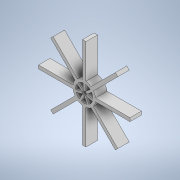
# Autodesk Inventor part: ЛОПАСТИ
Saved by Autodesk Inventor 2020 (Build 240168000, 168)
## iProperties
Created: 2020-09-18
Part Number: ЛОПАСТИ
Material: Типовые
Document SubType Name: Modeling
Designer: uchenik
Density: 1 g/cm^3
Appearance: По умолчанию
Author: uchenik
Autodesk Inventor part; units mm, degrees
ref_plane "YZ Plane" through (0, 0, 0) normal (1, 0, 0) x (0, 1, 0)
ref_plane "XZ Plane" through (0, 0, 0) normal (0, 1, 0) x (-1, 0, 0)
ref_plane "XY Plane" through (0, 0, 0) normal (0, 0, 1) x (1, 0, 0)
sketch "Эскиз1" plane through (0, 0, 0) normal (0, 0, 1) x (1, 0, 0)
  circle A0 centre (0, 0) radius 40
  circle A1 centre (0, 0) radius 10
  circle A2 centre (0, 0) radius 7.5
  line L0 (-1.5, 7.3485) -> (-1.5, 39.9719)
  line L1 (1.5, 7.3485) -> (1.5, 39.9719)
  line L2 (-6.2568, 4.1355) -> (-29.325, 27.2037)
  line L3 (-4.1355, 6.2568) -> (-27.2037, 29.325)
  line L4 (-7.3485, -1.5) -> (-39.9719, -1.5)
  line L5 (-7.3485, 1.5) -> (-39.9719, 1.5)
  line L6 (-4.1355, -6.2568) -> (-27.2037, -29.325)
  line L7 (-6.2568, -4.1355) -> (-29.325, -27.2037)
  line L8 (1.5, -7.3485) -> (1.5, -39.9719)
  line L9 (-1.5, -7.3485) -> (-1.5, -39.9719)
  line L10 (6.2568, -4.1355) -> (29.325, -27.2037)
  line L11 (4.1355, -6.2568) -> (27.2037, -29.325)
  line L12 (7.3485, 1.5) -> (39.9719, 1.5)
  line L13 (7.3485, -1.5) -> (39.9719, -1.5)
  line L14 (4.1355, 6.2568) -> (27.2037, 29.325)
  line L15 (6.2568, 4.1355) -> (29.325, 27.2037)
  circle A3 centre (0, 0) radius 2
  line L16 (-0.8877, 1.7922) -> (-0.8877, 7.4473)
  line L17 (0.8877, 1.7922) -> (0.8877, 7.4473)
  line L18 (-1.9547, 0.4233) -> (-6.376, 3.9492)
  line L19 (-0.8477, 1.8115) -> (-5.269, 5.3374)
  line L20 (-1.5497, -1.2643) -> (-7.063, -2.5227)
  line L21 (-1.9448, 0.4667) -> (-7.4581, -0.7917)
  line L22 (0.0222, -1.9999) -> (-2.4314, -7.0949)
  line L23 (-1.5774, -1.2295) -> (-4.0311, -6.3246)
  line L24 (1.5774, -1.2295) -> (4.0311, -6.3246)
  line L25 (-0.0222, -1.9999) -> (2.4314, -7.0949)
  line L26 (1.9448, 0.4667) -> (7.4581, -0.7917)
  line L27 (1.5497, -1.2643) -> (7.063, -2.5227)
  line L28 (0.8477, 1.8115) -> (5.269, 5.3374)
  line L29 (1.9547, 0.4233) -> (6.376, 3.9492)
  circle A4 centre (-0.0222, 0) radius 1.75
  point P0 (0, 7.5)
  point P1 (-1.5, 9.8869)
  point P2 (-5.9304, 8.0517)
  point P3 (-8.0517, 5.9304)
  point P4 (-9.8869, 1.5)
  point P5 (-9.8869, -1.5)
  point P6 (-8.0517, -5.9304)
  point P7 (-5.9304, -8.0517)
  point P8 (-1.5, -9.8869)
  point P9 (1.5, -9.8869)
  point P10 (5.9304, -8.0517)
  point P11 (8.0517, -5.9304)
  point P12 (9.8869, -1.5)
  point P13 (9.8869, 1.5)
  point P14 (8.0517, 5.9304)
  point P15 (27.2037, 29.325)
  point P16 (5.9304, 8.0517)
  point P17 (1.5, 9.8869)
  point P18 (1.9947, 0.4553)
  point P19 (1.5996, -1.2757)
  point P20 (7.4581, -0.7917)
  point P21 (0.8877, 1.8434)
  point P22 (0, -2.046)
  point P23 (-1.5996, -1.2757)
  point P24 (-1.9947, 0.4553)
  point P25 (-0.8877, 1.8434)
  dimension "d3" = 80
  dimension "d4" = 20
  dimension "d5" = 15
  dimension "d6" = 3
  dimension "d7" = 1.5
  dimension "d8" = 1.5
  dimension "d11" = 360
  dimension "d15" = 4
  dimension "d18" = 360
  dimension "d20" = 3.5
  constraints: 60 end point, 9 point on circle, 5 centre point, 4 coincident, 2 parallel, 2 vertical, 92 other
  measures "d3" diameter of A0
  measures "d4" diameter of A1
  measures "d5" diameter of A2
  measures "d6" distance between parallel lines of L0 L1
  measures "d7" distance from line of point (0, 7.5) L0
  measures "d8" distance from line of point (0, 7.5) L1
  measures "d15" diameter of A3
  measures "d20" diameter of A4
extrude "Выдавливание1" add sketch "Эскиз1" along normal blind 10 contours A0 L13 A1 L12 | L15 A1 L14 A0 | L12 A2 L15 A1 | A1 L13 A2 L12 | A0 L11 A1 L10 | A1 L10 A2 L13 | L15 A2 L14 A1 | A1 L11 A2 L10 | A2 L27 L24 A3 L29 L26 | L1 A1 L0 A0 | L14 A2 L1 A1 | A2 L29 L26 A3 L17 L28 | A0 L9 A1 L8 | A1 L8 A2 L11 | L1 A2 L0 A1 | A1 L9 A2 L8 | L24 A2 L25 L22 A3 L27 | L3 A1 L2 A0 | L0 A2 L3 A1 | L28 A3 L19 L16 A2 L17 | A3 | A0 L7 A1 L6 | A1 L6 A2 L9 | L3 A2 L2 A1 | A1 L7 A2 L6 | L5 A1 L4 A0 | L2 A2 L5 A1 | A1 L4 A2 L7 | A2 L23 L20 A3 L25 L22 | L5 A2 L4 A1 | A2 L19 L16 A3 L21 L18 | A2 L21 L18 A3 L23 L20
equation "\"d7\" = d8"
